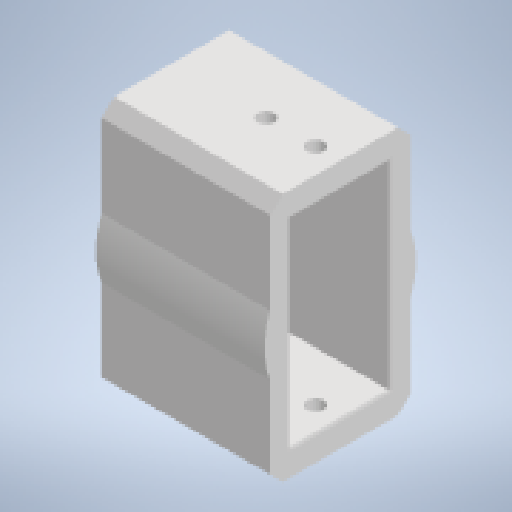
# Autodesk Inventor part: connectpart1
Saved by Autodesk Inventor 2024.3 (Build 283343010, 343A)
## iProperties
Created: 2025-06-26
Part Number: connectpart1
Material: 一般
Document SubType Name: Modeling
Designer: kshau
Density: 1 g/cm^3
Appearance: 既定
Mass: 20.286 g
Surface Area: 105.021 cm^2
Volume: 20.286 cm^3
Author: kshau
Autodesk Inventor part; units mm, degrees
ref_plane "YZ Plane" through (0, 0, 0) normal (1, 0, 0) x (0, 1, 0)
ref_plane "XZ Plane" through (0, 0, 0) normal (0, 1, 0) x (-1, 0, 0)
ref_plane "XY Plane" through (0, 0, 0) normal (0, 0, 1) x (1, 0, 0)
sketch "スケッチ1" plane through (0, 0, 0) normal (1, 0, 0) x (0, 1, 0)
  line L0 (0, 0) -> (50.2, 0)
  line L1 (50.2, 0) -> (50.2, -28.2)
  line L2 (50.2, -28.2) -> (0, -28.2)
  line L3 (0, -28.2) -> (0, 0)
  line L4 (50.2, -14.1) -> (0, -14.1)
  line L5 (25.1, -28.2) -> (25.1, 0)
  circle A0 centre (25.1, -14.1) radius 15.3335
  point P0 (19.0745, 0)
  point P1 (19.0745, -28.2)
  point P2 (31.1255, -28.2)
  point P3 (31.1255, 0)
  dimension "d0" = 50.2
  dimension "d1" = 28.2
  dimension "d2" = 30.667
  constraints: 12 end point, 5 midpoint, 2 parallel, 1 centre point, 1 horizontal, 1 perpendicular
  measures "d0" distance of L1.end L2.end
  measures "d1" distance of L2.end L0.start
  measures "d2" diameter of A0
extrude "押し出し1" add sketch "スケッチ1" against normal blind 34
chamfer "面取り1" distance 2.5 angle 45 4 edges at (-17, 50.2, 0) (-17, 50.2, -28.2) (-17, 0, 0) (-17, 0, -28.2)
sketch "スケッチ2" plane through (-34, 0, 0) normal (-1, 0, 0) x (0, 0, 1)
  arc A0 (-28.2, 31.1255) -> (-28.2, 19.0745) centre (-14.1, 25.1) ccw projected
  circle A1 centre (-14.1, 25.1) radius 19.5
  point P0 (0, 0)
  dimension "d8" = 39
  constraints: 1 centre point, 1 coincident
  measures "d8" diameter of A1
extrude "押し出し2" [suppressed]
sketch "スケッチ3" plane through (-36.375, 22.6, -13.1) normal (-1, 0, 0) x (0, 0, 1)
  arc A0 (-13.1, -14.4444) -> (13.1, -14.4444) centre (0, 0) ccw projected
  circle A1 centre (0, 0) radius 23
  point P0 (13.1, -22.6)
  dimension "d11" = 46
  constraints: 1 centre point, 1 coincident
  measures "d11" diameter of A1
extrude "押し出し3" [suppressed]
sketch "スケッチ4" plane through (-42.675, 22.6, -13.1) normal (-1, 0, 0) x (0, 0, 1)
  circle A0 centre (0, 0) radius 23 projected
  line L0 (0, 0) -> (19.85, 0)
  line L1 (19.85, 0) -> (19.85, 16.35)
  line L2 (19.85, 16.35) -> (0, 16.35)
  line L3 (0, 16.35) -> (0, 0)
  line L4 (10.6, 22.6) -> (-10.6, 22.6) projected
  line L5 (19.85, 0) -> (0, 0)
  line L6 (0, 0) -> (0, -14.35)
  line L7 (0, -14.35) -> (19.85, -14.35)
  line L8 (19.85, -14.35) -> (19.85, 0)
  line L9 (-19.85, 0) -> (-19.85, 16.35)
  line L10 (-19.85, 16.35) -> (0, 16.35)
  line L11 (0, -14.35) -> (-19.85, -14.35)
  line L12 (-19.85, -14.35) -> (-19.85, 0)
  point P0 (13.1, -22.6)
  point P1 (17.9744, -14.35)
  point P2 (19.85, -11.618)
  point P3 (19.85, 11.618)
  point P4 (16.1764, 16.35)
  point P5 (-16.1764, 16.35)
  point P6 (-19.85, 11.618)
  point P7 (-19.85, -11.618)
  point P8 (-17.9744, -14.35)
  dimension "d14" = 6.25
  dimension "d16" = 19.85
  dimension "d17" = 30.7
  constraints: 24 end point, 4 parallel, 3 symmetric about line, 2 horizontal, 2 perpendicular
  measures "d14" distance between parallel lines of L4 L2
  measures "d16" distance between parallel lines of L3 L1
  measures "d17" distance between parallel lines of L2 L7
extrude "押し出し4" [suppressed]
sketch "スケッチ5" plane through (-47.675, 22.6, -13.1) normal (-1, 0, 0) x (0, 0, 1)
  line L0 (-16.1764, 16.35) -> (16.1764, 16.35) projected
  line L1 (0, 16.35) -> (0, -14.35)
  line L2 (17.9744, -14.35) -> (-17.9744, -14.35) projected
  line L3 (0, -14.35) -> (16.75, -14.35)
  line L4 (16.75, -14.35) -> (16.75, 13.35)
  line L5 (16.75, 13.35) -> (0, 13.35)
  line L6 (0, 13.35) -> (0, -14.35)
  line L7 (19.85, -11.618) -> (19.85, 11.618) projected
  line L8 (-16.75, -14.35) -> (-16.75, 13.35)
  line L9 (-16.75, 13.35) -> (0, 13.35)
  point P0 (13.1, -22.6)
  point P1 (19.85, -14.35)
  point P2 (19.85, 16.35)
  point P3 (-16.75, -14.35)
  dimension "d20" = 3
  dimension "d21" = 3.1
  constraints: 14 end point, 2 midpoint, 2 parallel, 2 symmetric about line, 1 horizontal, 1 perpendicular
  measures "d20" distance between parallel lines of L0 L5
  measures "d21" distance between parallel lines of L7 L4
extrude "押し出し5" [suppressed]
sketch "スケッチ6" plane through (0, 0, 0) normal (1, 0, 0) x (0, 0, -1)
  line L0 (2.5, 50.2) -> (25.7, 50.2) projected
  line L1 (14.1, 50.2) -> (14.1, 0)
  line L2 (2.5, 0) -> (25.7, 0) projected
  arc A0 (0, 31.1255) -> (0, 19.0745) centre (14.1, 25.1) ccw projected
  line L3 (14.1, 25.1) -> (29.4335, 25.1)
  arc A1 (28.2, 19.0745) -> (28.2, 31.1255) centre (14.1, 25.1) ccw projected
  line L4 (14.1, 25.1) -> (24.2, 25.1)
  line L5 (24.2, 25.1) -> (24.2, 45.2)
  line L6 (24.2, 45.2) -> (14.1, 45.2)
  line L7 (14.1, 45.2) -> (14.1, 25.1)
  line L8 (24.2, 25.1) -> (24.2, 5)
  line L9 (24.2, 5) -> (14.1, 5)
  line L10 (4, 25.1) -> (4, 45.2)
  line L11 (4, 45.2) -> (14.1, 45.2)
  line L12 (4, 5) -> (14.1, 5)
  line L13 (4, 25.1) -> (4, 5)
  point P0 (0, 0)
  dimension "d24" = 20.1
  dimension "d25" = 10.1
  constraints: 24 end point, 5 symmetric about line, 2 horizontal, 2 midpoint, 2 parallel, 1 perpendicular, 1 point on circle
  measures "d24" distance of L4.end L5.end
  measures "d25" distance of L5.end L6.end
extrude "押し出し6" cut sketch "スケッチ6" against normal blind 25
sketch "スケッチ7" plane through (-42.675, 22.6, -13.1) normal (-1, 0, 0) x (0, 0, 1)
  circle A0 centre (0, -0.4) radius 13
  line L0 (-16.75, 13.35) -> (16.75, 13.35) projected
  line L1 (0, 13.35) -> (0, -0.4)
  point P0 (13.1, -22.6)
  dimension "d28" = 26
  dimension "d29" = 13.75
  constraints: 2 end point, 1 centre point, 1 midpoint, 1 vertical
  measures "d28" diameter of A0
  measures "d29" distance from line of L0 L1.end
extrude "押し出し7" [suppressed]
sketch "スケッチ8" plane through (-40.175, 22.2, -13.1) normal (-1, 0, 0) x (0, 0, 1)
  circle A0 centre (0, 0) radius 5
  point P0 (13.1, -22.2)
  dimension "d32" = 10
  constraints: 1 centre point
  measures "d32" diameter of A0
extrude "押し出し8" [suppressed]
sketch "スケッチ9" plane through (-40.175, 22.2, -13.1) normal (-1, 0, 0) x (0, 0, 1)
  circle A0 centre (0, 0) radius 11
  circle A1 centre (0, 0) radius 13 projected
  point P0 (13.1, -22.2)
  point P1 (0, 11)
  point P2 (-7.7782, 7.7782)
  point P3 (-11, 0)
  point P4 (-7.7782, -7.7782)
  point P5 (0, -11)
  point P6 (7.7782, -7.7782)
  point P7 (11, 0)
  point P8 (7.7782, 7.7782)
  dimension "d35" = 22
  dimension "d38" = 360
  constraints: 1 vertical alignment, 12 other
hole "穴1" [suppressed]
sketch "スケッチ11" plane through (-37.875, 22.2, -13.1) normal (-1, 0, 0) x (0, 0, 1)
  circle A0 centre (0, 0) radius 5 projected
  point P0 (13.1, -22.2)
  constraints: 1 coincident
hole "穴2" [suppressed]
sketch "スケッチ12" plane through (-25, 0, 0) normal (1, 0, 0) x (0, 0, -1)
  circle A0 centre (13.1, 22.2) radius 1.55 projected
  circle A1 centre (13.1, 22.2) radius 3
  point P0 (0, 0)
  dimension "d57" = 6
  constraints: 1 centre point, 1 coincident
  measures "d57" diameter of A1
extrude "押し出し10" [suppressed]
sketch "スケッチ13" plane through (-25, 0, 0) normal (1, 0, 0) x (0, 0, -1)
  circle A0 centre (5.3218, 29.9782) radius 1.25 projected
  circle A1 centre (5.3218, 29.9782) radius 2.25
  circle A2 centre (20.8782, 29.9782) radius 1.25 projected
  circle A3 centre (20.8782, 29.9782) radius 2.25
  circle A4 centre (5.3218, 14.4218) radius 1.25 projected
  circle A5 centre (5.3218, 14.4218) radius 2.25
  circle A6 centre (20.8782, 14.4218) radius 1.25 projected
  circle A7 centre (20.8782, 14.4218) radius 2.25
  point P0 (0, 0)
  dimension "d60" = 4.5
  dimension "d61" = 4.5
  dimension "d62" = 4.5
  dimension "d63" = 4.5
  constraints: 4 centre point, 4 coincident
  measures "d60" diameter of A1
  measures "d61" diameter of A3
  measures "d62" diameter of A5
  measures "d63" diameter of A7
extrude "押し出し11" [suppressed]
sketch "スケッチ14" plane through (-25, 0, 0) normal (1, 0, 0) x (0, 0, -1)
  line L0 (4, 45.2) -> (24.2, 45.2) projected
  line L1 (14.1, 45.2) -> (14.1, 5)
  line L2 (24.2, 5) -> (4, 5) projected
  point P0 (0, 0)
  point P1 (14.1, 15.1)
  point P2 (14.1, 25.1)
  point P3 (14.1, 35.1)
  dimension "d66" = 10
  dimension "d67" = 10
  constraints: 3 midpoint, 2 end point, 2 point on line
  measures "d66" distance of point (14.1, 15.1) point (14.1, 25.1)
  measures "d67" distance of point (14.1, 25.1) point (14.1, 35.1)
hole "穴3" [suppressed]
sketch "スケッチ15" plane through (-40.175, 22.2, -13.1) normal (-1, 0, 0) x (0, 0, 1)
  point P0 (13.1, -22.2)
sketch "スケッチ16" plane through (-34, 0, 0) normal (-1, 0, 0) x (0, 0, 1)
  arc A0 (-28.2, 31.1255) -> (-28.2, 19.0745) centre (-14.1, 25.1) ccw projected
  circle A1 centre (-14.1, 25.1) radius 11
  point P0 (0, 0)
  point P1 (-14.1, 36.1)
  point P2 (-6.3218, 32.8782)
  point P3 (-3.1, 25.1)
  point P4 (-6.3218, 17.3218)
  point P5 (-14.1, 14.1)
  point P6 (-21.8782, 17.3218)
  point P7 (-25.1, 25.1)
  point P8 (-21.8782, 32.8782)
  dimension "d75" = 22
  dimension "d78" = 360
  constraints: 1 coincident, 1 vertical alignment, 11 other
hole "穴4" at (-34, 32.8782, -21.8782) at (-34, 36.1, -14.1) at (-34, 32.8782, -6.3218) at (-34, 17.3218, -6.3218) at (-34, 14.1, -14.1) at (-34, 17.3218, -21.8782) direction (1, 0, 0) diameter 2.7 end through all
sketch "スケッチ17" plane through (-25, 0, 0) normal (1, 0, 0) x (0, 0, -1)
  circle A0 centre (14.1, 36.1) radius 1.35 projected
  circle A1 centre (6.3218, 32.8782) radius 1.35 projected
  circle A2 centre (21.8782, 32.8782) radius 1.35 projected
  circle A3 centre (21.8782, 17.3218) radius 1.35 projected
  circle A4 centre (14.1, 14.1) radius 1.35 projected
  circle A5 centre (6.3218, 17.3218) radius 1.35 projected
  point P0 (0, 0)
  constraints: 6 coincident
hole "穴5" at (-25, 36.1, -14.1) at (-25, 32.8782, -6.3218) at (-25, 32.8782, -21.8782) at (-25, 17.3218, -21.8782) at (-25, 14.1, -14.1) at (-25, 17.3218, -6.3218) direction (-1, 0, 0) diameter 4.9 depth 2.6
sketch "スケッチ18" plane through (0, 0, -25.7) normal (0, -1, 0) x (1, 0, 0)
  line L0 (-34, 0) -> (0, 0) projected
  line L1 (-15, 0) -> (-15, 23.2)
  line L2 (0, 23.2) -> (-34, 23.2) projected
  line L3 (-25, 1.5) -> (-25, 21.7) projected
  line L4 (-5, 0) -> (-5, 23.2)
  line L5 (-5, 11.6) -> (-15, 11.6)
  point P0 (0, 25.7)
  dimension "d94" = 10
  dimension "d95" = 10
  constraints: 6 end point, 4 point on line, 2 coincident, 2 midpoint, 1 perpendicular, 1 vertical
  measures "d94" distance between parallel lines of L3 L1
  measures "d95" distance between parallel lines of L1 L4
hole "穴6" at (-15, 0, -14.1) at (-5, 0, -14.1) direction (0, 1, 0) diameter 3.3 end through all
fillet "フィレット1" radius 0.5 4 edges at (0, 45.2, -14.1) (0, 25.1, -4) (0, 25.1, -24.2) (0, 5, -14.1)
